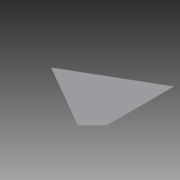
# Autodesk Inventor part: Triangle
Saved by Autodesk Inventor 2016 (Build 200138000, 138)
## iProperties
Created: 2016-02-24
Part Number: Triangle
Material: Generic
Document SubType Name: Modeling
Designer: jonesdm
Density: 1 g/cm^3
Appearance: Default
Author: jonesdm
Autodesk Inventor part; units mm, degrees
ref_plane "YZ Plane" through (0, 0, 0) normal (1, 0, 0) x (0, 1, 0)
ref_plane "XZ Plane" through (0, 0, 0) normal (0, 1, 0) x (-1, 0, 0)
ref_plane "XY Plane" through (0, 0, 0) normal (0, 0, 1) x (1, 0, 0)
sketch "Sketch1" plane through (0, 0, 0) normal (0, 1, 0) x (-1, 0, 0)
  line L0 (-923.8759, 1066.8) -> (-923.8759, -1066.8)
  line L1 (-923.8759, -1066.8) -> (923.8759, 0)
  line L2 (-923.8759, 1066.8) -> (923.8759, 0)
  point P0 (0, 0)
  point P1 (0, -533.4)
  dimension "d2" = 2133.6
  constraints: 6 end point, 2 equal length, 1 horizontal alignment, 1 midpoint, 1 vertical, 1 vertical alignment
  measures "d2" distance of L0.end L1.end
extrude "Extrusion1" add sketch "Sketch1" along normal blind 0.508
body "Solid1"
